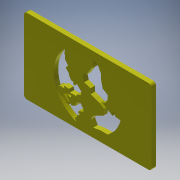
# Autodesk Inventor part: kaart
Saved by Autodesk Inventor 2019 (Build 230136000, 136)
## iProperties
Created: 2020-06-08
Part Number: kaart
Material: Generic
Document SubType Name: Modeling
Designer: Jaap Kort
Density: 1 g/cm^3
Appearance: Yellow
Author: Jaap Kort
Autodesk Inventor part; units mm, degrees
ref_plane "YZ Plane" through (0, 0, 0) normal (1, 0, 0) x (0, 1, 0)
ref_plane "XZ Plane" through (0, 0, 0) normal (0, 1, 0) x (-1, 0, 0)
ref_plane "XY Plane" through (0, 0, 0) normal (0, 0, 1) x (1, 0, 0)
sketch "Sketch1" plane through (0, 0, 0) normal (0, 0, 1) x (1, 0, 0)
  line L0 (42.5, 25) -> (-42.5, 25)
  line L1 (-42.5, 25) -> (-42.5, -25)
  line L2 (-42.5, -25) -> (42.5, -25)
  line L3 (42.5, -25) -> (42.5, 25)
  line L4 (42.5, 25) -> (-42.5, -25) construction
  line L5 (-42.5, 25) -> (42.5, -25) construction
  point P0 (0, 0)
  dimension "d5" = 85
  dimension "d6" = 50
  constraints: 12 end point, 2 midpoint, 2 parallel, 1 horizontal, 1 perpendicular
  measures "d5" distance of L2.end L1.end
  measures "d6" distance of L1.end L0.end
extrude "Extrusion1" add sketch "Sketch1" along normal blind 3
fillet "Fillet1" radius 2 4 edges at (-42.5, 25, 1.5) (-42.5, -25, 1.5) (42.5, 25, 1.5) (42.5, -25, 1.5)
sketch "Sketch3" plane through (0, 0, 3) normal (0, 0, 1) x (1, 0, 0)
  line L0 (10.1884, -9.0431) -> (3.6225, -12.2145) projected
  line L1 (3.6225, -12.2145) -> (1.8471, -15.4815) projected
  line L2 (1.8471, -15.4815) -> (3.6225, -19.1574) projected
  line L3 (3.6225, -19.1574) -> (8.4303, -18.306) projected
  line L4 (8.4303, -18.306) -> (13.3598, -18.306) projected
  arc A0 (13.3598, -18.306) -> (21.8774, -5.9135) centre (0.0004, -0.0005) ccw projected
  line L5 (21.8774, -5.9135) -> (18.3227, -5.4251) projected
  line L6 (18.3227, -5.4251) -> (17.7172, -3.3976) projected
  line L7 (17.7172, -3.3976) -> (16.2771, -3.9611) projected
  line L8 (16.2771, -3.9611) -> (16.4595, -5.9135) projected
  line L9 (16.4595, -5.9135) -> (9.6956, -1.8296) projected
  line L10 (9.6956, -1.8296) -> (11.7603, -0.7368) projected
  line L11 (11.7603, -0.7368) -> (13.3756, 1.9385) projected
  line L12 (13.3756, 1.9385) -> (13.3756, 4.441) projected
  line L13 (13.3756, 4.441) -> (9.9852, 6.488) projected
  line L14 (9.9852, 6.488) -> (8.7469, 11.5278) projected
  line L15 (10.8087, -4.6996) -> (10.1884, -9.0431) projected
  line L16 (7.8248, -2.8198) -> (10.8087, -4.6996) projected
  line L17 (5.0084, -1.7547) -> (7.8248, -2.8198) projected
  line L18 (1.847, -0.7368) -> (5.0084, -1.7547) projected
  line L19 (1.847, 2.6578) -> (1.847, -0.7368) projected
  line L20 (-2.3849, 4.0204) -> (1.847, 2.6578) projected
  line L21 (-3.2331, 7.4725) -> (-2.3849, 4.0204) projected
  line L22 (-3.2331, 9.173) -> (-3.2331, 7.4725) projected
  line L23 (-0.8369, 9.173) -> (-3.2331, 9.173) projected
  line L24 (2.6285, 14.9126) -> (-0.8369, 9.173) projected
  line L25 (3.7858, 15.5252) -> (2.6285, 14.9126) projected
  line L26 (3.7858, 17.0153) -> (3.7858, 15.5252) projected
  line L27 (3.0996, 19.808) -> (3.7858, 17.0153) projected
  line L28 (6.2699, 19.3552) -> (3.0996, 19.808) projected
  line L29 (8.7469, 14.6753) -> (6.2699, 19.3552) projected
  line L30 (8.7469, 11.5278) -> (8.7469, 14.6753) projected
  line L31 (-15.5454, 14.131) -> (-15.1575, 16.8475) projected
  arc A1 (-15.1575, 16.8475) -> (-21.3544, -7.5881) centre (0, 0) ccw projected
  line L32 (-15.1575, 13.1395) -> (-15.5454, 14.131) projected
  line L33 (-15.1575, 10.8024) -> (-15.1575, 13.1395) projected
  line L34 (-13.5038, 8.9132) -> (-15.1575, 10.8024) projected
  line L35 (-13.1136, 7.916) -> (-13.5038, 8.9132) projected
  line L36 (-14.7449, 6.488) -> (-13.1136, 7.916) projected
  line L37 (-12.4652, 3.8837) -> (-14.7449, 6.488) projected
  line L38 (-12.5717, 3.1381) -> (-12.4652, 3.8837) projected
  line L39 (-11.0213, 0.739) -> (-12.5717, 3.1381) projected
  line L40 (-9.7126, 0.739) -> (-11.0213, 0.739) projected
  line L41 (-9.7126, -0.776) -> (-9.7126, 0.739) projected
  line L42 (-8.3865, -0.776) -> (-9.7126, -0.776) projected
  line L43 (-7.4718, 0.739) -> (-8.3865, -0.776) projected
  line L44 (-4.3285, -2.2451) -> (-7.4718, 0.739) projected
  line L45 (-4.4825, -4.4433) -> (-4.3285, -2.2451) projected
  line L46 (-7.4718, -5.671) -> (-4.4825, -4.4433) projected
  line L47 (-7.545, -6.7157) -> (-7.4718, -5.671) projected
  line L48 (-10.0699, -6.5388) -> (-7.545, -6.7157) projected
  line L49 (-11.9728, -6.7157) -> (-10.0699, -6.5388) projected
  line L50 (-12.4652, -4.8389) -> (-11.9728, -6.7157) projected
  line L51 (-15.9878, -4.5571) -> (-12.4652, -4.8389) projected
  line L52 (-15.569, -6.1534) -> (-15.9878, -4.5571) projected
  line L53 (-18.4139, -5.954) -> (-15.569, -6.1534) projected
  line L54 (-19.7745, -6.7102) -> (-18.4139, -5.954) projected
  line L55 (-19.9068, -8.7509) -> (-19.7745, -6.7102) projected
  arc A2 (-21.3544, -7.5881) -> (-19.8841, -10.8724) centre (0, 0) ccw projected
  arc A3 (-19.8841, -10.8724) -> (-7.6172, -21.344) centre (0, 0) ccw projected
  line L56 (-19.3329, -10.004) -> (-19.9068, -8.7509) projected
  line L57 (-18.4139, -11.1806) -> (-19.3329, -10.004) projected
  line L58 (-16.9914, -11.4788) -> (-18.4139, -11.1806) projected
  line L59 (-15.7885, -11.4788) -> (-16.9914, -11.4788) projected
  line L60 (-14.5622, -12.8854) -> (-15.7885, -11.4788) projected
  line L61 (-16.4001, -9.4308) -> (-13.0579, -12.7288) projected
  line L62 (-16.0242, -9.0499) -> (-16.4001, -9.4308) projected
  line L63 (-15.6483, -9.4208) -> (-16.0242, -9.0499) projected
  line L64 (-14.73, -8.4902) -> (-15.6483, -9.4208) projected
  line L65 (-12.5087, -7.815) -> (-14.668, -8.4658) projected
  line L66 (-11.5048, -7.815) -> (-12.5087, -7.815) projected
  line L67 (-10.9029, -8.2239) -> (-11.5048, -7.815) projected
  line L68 (-11.5049, -9.11) -> (-10.9029, -8.2239) projected
  line L69 (-12.8585, -9.11) -> (-11.5049, -9.11) projected
  line L70 (-14.668, -8.4658) -> (-14.73, -8.4902) projected
  line L71 (-13.9227, -9.3449) -> (-13.0966, -8.875) projected
  line L72 (-13.0966, -8.875) -> (-12.8585, -9.11) projected
  line L73 (-11.5072, -12.1943) -> (-13.9227, -9.3449) projected
  line L74 (-14.5622, -13.8641) -> (-14.5622, -12.8854) projected
  line L75 (-12.61, -13.8641) -> (-14.5622, -13.8641) projected
  line L76 (-13.0579, -12.7288) -> (-12.61, -13.8641) projected
  line L77 (-11.0213, -13.5896) -> (-11.5072, -12.1943) projected
  line L78 (-10.3243, -13.5896) -> (-11.0213, -13.5896) projected
  line L79 (-9.3697, -12.7803) -> (-10.3243, -13.5896) projected
  line L80 (-8.4588, -12.7803) -> (-9.3697, -12.7803) projected
  line L81 (-7.8216, -10.6631) -> (-8.4588, -12.7803) projected
  line L82 (-6.3597, -9.3449) -> (-7.8216, -10.6631) projected
  line L83 (-4.5047, -9.3449) -> (-6.3597, -9.3449) projected
  line L84 (-3.9638, -10.3994) -> (-4.5047, -9.3449) projected
  line L85 (-2.9667, -11.3833) -> (-3.9638, -10.3994) projected
  line L86 (-2.9667, -13.3007) -> (-2.9667, -11.3833) projected
  line L87 (-6.3787, -14.6467) -> (-2.9667, -13.3007) projected
  line L88 (-6.1868, -14.6467) -> (-6.3787, -14.6467) projected
  line L89 (-6.1868, -15.6933) -> (-6.1868, -14.6467) projected
  line L90 (-5.4322, -15.6933) -> (-6.1868, -15.6933) projected
  line L91 (-5.5915, -16.8087) -> (-5.4322, -15.6933) projected
  line L92 (-6.3597, -16.8087) -> (-5.5915, -16.8087) projected
  arc A4 (-6.3597, -16.8087) -> (-7.2455, -18.052) centre (-5.9895, -18.0096) ccw projected
  arc A5 (-8.4619, -18.9525) -> (-7.2455, -18.052) centre (-8.164, -18.0831) ccw projected
  line L93 (-8.4619, -19.8829) -> (-8.4619, -18.9525) projected
  line L94 (-7.6172, -21.344) -> (-8.4619, -19.8829) projected
  line L95 (-6.2198, -19.1959) -> (-6.2198, -19.828) projected
  line L96 (-5.6245, -18.1685) -> (-6.2198, -19.1959) projected
  line L97 (-4.6572, -17.6144) -> (-5.6245, -18.1685) projected
  line L98 (-4.0769, -17.6144) -> (-4.6572, -17.6144) projected
  line L99 (-3.4652, -17.9689) -> (-4.0769, -17.6144) projected
  line L100 (-3.4652, -18.6822) -> (-3.4652, -17.9689) projected
  line L101 (-4.3582, -18.6822) -> (-3.4652, -18.6822) projected
  line L102 (-5.0222, -19.828) -> (-4.3582, -18.6822) projected
  line L103 (-5.6245, -20.173) -> (-5.0222, -19.828) projected
  line L104 (-6.2198, -19.828) -> (-5.6245, -20.173) projected
  point P0 (0, 0)
  constraints: 1 other
extrude "Extrusion2" cut sketch "Sketch3" against normal blind 0.6 contours L15 L16 L17 L18 L19 L20 L21 L22 L23 L24 L25 L26 L27 L28 L29 L30 L14 L13 L12 L11 L10 L9 L8 L7 L6 L5 A0 L4 L3 L2 L1 L0 | L32 L33 L34 L35 L36 L37 L38 L39 L40 L41 L42 L43 L44 L45 L46 L47 L48 L49 L50 L51 L52 L53 L54 L55 L56 L57 L58 L59 L60 L74 L75 L76 L61 L62 L63 L64 L70 L65 L66 L67 L68 L69 L72 L71 L73 L77 L78 L79 L80 L81 L82 L83 L84 L85 L86 L87 L88 L89 L90 L91 L92 A4 A5 L93 L94 A3 A2 A1 L31
body "Solid1"
